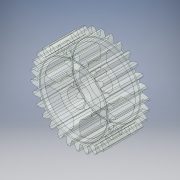
# Autodesk Inventor part: Peça1
Saved by Autodesk Inventor 2019.4 (Build 234330000, 330)
## iProperties
Created: 2020-04-11
Part Number: Peça1
Material: Vidro, fundido, transparente
Document SubType Name: Modeling
Designer: lucas
Density: 2.18 g/cm^3
Appearance: Transparente
Author: lucas
Autodesk Inventor part; units mm, degrees
ref_plane "YZ Plane" through (0, 0, 0) normal (1, 0, 0) x (0, 1, 0)
ref_plane "XZ Plane" through (0, 0, 0) normal (0, 1, 0) x (-1, 0, 0)
ref_plane "XY Plane" through (0, 0, 0) normal (0, 0, 1) x (1, 0, 0)
sketch "Esboço1" plane through (0, 0, 0) normal (0, 0, 1) x (1, 0, 0)
  circle A0 centre (0, 0) radius 35 construction
  arc A1 (-1.094, 31.8562) -> (-3.3459, 37.3504) centre (-14.2896, 29.6565) ccw
  arc A2 (3.3459, 37.3504) -> (1.094, 31.8562) centre (14.2896, 29.6565) ccw
  arc A3 (1.094, 31.8562) -> (-1.094, 31.8562) centre (0, 0) ccw
  arc A4 (6.0221, 31.301) -> (5.0493, 37.1585) centre (-7.3322, 32.0927) ccw
  arc A5 (8.1553, 30.8141) -> (6.0221, 31.301) centre (0, 0) ccw
  arc A6 (11.5732, 35.6695) -> (8.1553, 30.8141) centre (20.5306, 25.7332) ccw
  arc A7 (12.8362, 29.1762) -> (13.1912, 35.1033) centre (-0.007, 32.9196) ccw
  arc A8 (14.8076, 28.2268) -> (12.8362, 29.1762) centre (0, 0) ccw
  arc A9 (19.2203, 32.1999) -> (14.8076, 28.2268) centre (25.742, 20.5196) ccw
  arc A10 (19.0067, 25.5883) -> (20.6717, 31.2879) centre (7.3185, 32.0958) ccw
  arc A11 (20.7174, 24.2241) -> (19.0067, 25.5883) centre (0, 0) ccw
  arc A12 (25.9035, 27.1156) -> (20.7174, 24.2241) centre (29.6626, 14.277) ccw
  arc A13 (24.2241, 20.7174) -> (27.1156, 25.9035) centre (14.277, 29.6626) ccw
  arc A14 (25.5883, 19.0067) -> (24.2241, 20.7174) centre (0, 0) ccw
  arc A15 (31.2879, 20.6717) -> (25.5883, 19.0067) centre (32.0958, 7.3185) ccw
  arc A16 (28.2268, 14.8076) -> (32.1999, 19.2203) centre (20.5196, 25.742) ccw
  arc A17 (29.1762, 12.8362) -> (28.2268, 14.8076) centre (0, 0) ccw
  arc A18 (35.1033, 13.1912) -> (29.1762, 12.8362) centre (32.9196, -0.007) ccw
  arc A19 (30.8141, 8.1553) -> (35.6695, 11.5732) centre (25.7332, 20.5306) ccw
  arc A20 (31.301, 6.0221) -> (30.8141, 8.1553) centre (0, 0) ccw
  arc A21 (37.1585, 5.0493) -> (31.301, 6.0221) centre (32.0927, -7.3322) ccw
  arc A22 (31.8562, 1.094) -> (37.3504, 3.3459) centre (29.6565, 14.2896) ccw
  arc A23 (31.8562, -1.094) -> (31.8562, 1.094) centre (0, 0) ccw
  arc A24 (37.3504, -3.3459) -> (31.8562, -1.094) centre (29.6565, -14.2896) ccw
  arc A25 (31.301, -6.0221) -> (37.1585, -5.0493) centre (32.0927, 7.3322) ccw
  arc A26 (30.8141, -8.1553) -> (31.301, -6.0221) centre (0, 0) ccw
  arc A27 (35.6695, -11.5732) -> (30.8141, -8.1553) centre (25.7332, -20.5306) ccw
  arc A28 (29.1762, -12.8362) -> (35.1033, -13.1912) centre (32.9196, 0.007) ccw
  arc A29 (28.2268, -14.8076) -> (29.1762, -12.8362) centre (0, 0) ccw
  arc A30 (32.1999, -19.2203) -> (28.2268, -14.8076) centre (20.5196, -25.742) ccw
  arc A31 (25.5883, -19.0067) -> (31.2879, -20.6717) centre (32.0958, -7.3185) ccw
  arc A32 (24.2241, -20.7174) -> (25.5883, -19.0067) centre (0, 0) ccw
  arc A33 (27.1156, -25.9035) -> (24.2241, -20.7174) centre (14.277, -29.6626) ccw
  arc A34 (20.7174, -24.2241) -> (25.9035, -27.1156) centre (29.6626, -14.277) ccw
  arc A35 (19.0067, -25.5883) -> (20.7174, -24.2241) centre (0, 0) ccw
  arc A36 (20.6717, -31.2879) -> (19.0067, -25.5883) centre (7.3185, -32.0958) ccw
  arc A37 (14.8076, -28.2268) -> (19.2203, -32.1999) centre (25.742, -20.5196) ccw
  arc A38 (12.8362, -29.1762) -> (14.8076, -28.2268) centre (0, 0) ccw
  arc A39 (13.1912, -35.1033) -> (12.8362, -29.1762) centre (-0.007, -32.9196) ccw
  arc A40 (8.1553, -30.8141) -> (11.5732, -35.6695) centre (20.5306, -25.7332) ccw
  arc A41 (6.0221, -31.301) -> (8.1553, -30.8141) centre (0, 0) ccw
  arc A42 (5.0493, -37.1585) -> (6.0221, -31.301) centre (-7.3322, -32.0927) ccw
  arc A43 (1.094, -31.8562) -> (3.3459, -37.3504) centre (14.2896, -29.6565) ccw
  arc A44 (-1.094, -31.8562) -> (1.094, -31.8562) centre (0, 0) ccw
  arc A45 (-3.3459, -37.3504) -> (-1.094, -31.8562) centre (-14.2896, -29.6565) ccw
  arc A46 (-6.0221, -31.301) -> (-5.0493, -37.1585) centre (7.3322, -32.0927) ccw
  arc A47 (-8.1553, -30.8141) -> (-6.0221, -31.301) centre (0, 0) ccw
  arc A48 (-11.5732, -35.6695) -> (-8.1553, -30.8141) centre (-20.5306, -25.7332) ccw
  arc A49 (-12.8362, -29.1762) -> (-13.1912, -35.1033) centre (0.007, -32.9196) ccw
  arc A50 (-14.8076, -28.2268) -> (-12.8362, -29.1762) centre (0, 0) ccw
  arc A51 (-19.2203, -32.1999) -> (-14.8076, -28.2268) centre (-25.742, -20.5196) ccw
  arc A52 (-19.0067, -25.5883) -> (-20.6717, -31.2879) centre (-7.3185, -32.0958) ccw
  arc A53 (-20.7174, -24.2241) -> (-19.0067, -25.5883) centre (0, 0) ccw
  arc A54 (-25.9035, -27.1156) -> (-20.7174, -24.2241) centre (-29.6626, -14.277) ccw
  arc A55 (-24.2241, -20.7174) -> (-27.1156, -25.9035) centre (-14.277, -29.6626) ccw
  arc A56 (-25.5883, -19.0067) -> (-24.2241, -20.7174) centre (0, 0) ccw
  arc A57 (-31.2879, -20.6717) -> (-25.5883, -19.0067) centre (-32.0958, -7.3185) ccw
  arc A58 (-28.2268, -14.8076) -> (-32.1999, -19.2203) centre (-20.5196, -25.742) ccw
  arc A59 (-29.1762, -12.8362) -> (-28.2268, -14.8076) centre (0, 0) ccw
  arc A60 (-35.1033, -13.1912) -> (-29.1762, -12.8362) centre (-32.9196, 0.007) ccw
  arc A61 (-30.8141, -8.1553) -> (-35.6695, -11.5732) centre (-25.7332, -20.5306) ccw
  arc A62 (-31.301, -6.0221) -> (-30.8141, -8.1553) centre (0, 0) ccw
  arc A63 (-37.1585, -5.0493) -> (-31.301, -6.0221) centre (-32.0927, 7.3322) ccw
  arc A64 (-31.8562, -1.094) -> (-37.3504, -3.3459) centre (-29.6565, -14.2896) ccw
  arc A65 (-31.8562, 1.094) -> (-31.8562, -1.094) centre (0, 0) ccw
  arc A66 (-37.3504, 3.3459) -> (-31.8562, 1.094) centre (-29.6565, 14.2896) ccw
  arc A67 (-31.301, 6.0221) -> (-37.1585, 5.0493) centre (-32.0927, -7.3322) ccw
  arc A68 (-30.8141, 8.1553) -> (-31.301, 6.0221) centre (0, 0) ccw
  arc A69 (-35.6695, 11.5732) -> (-30.8141, 8.1553) centre (-25.7332, 20.5306) ccw
  arc A70 (-29.1762, 12.8362) -> (-35.1033, 13.1912) centre (-32.9196, -0.007) ccw
  arc A71 (-28.2268, 14.8076) -> (-29.1762, 12.8362) centre (0, 0) ccw
  arc A72 (-32.1999, 19.2203) -> (-28.2268, 14.8076) centre (-20.5196, 25.742) ccw
  arc A73 (-25.5883, 19.0067) -> (-31.2879, 20.6717) centre (-32.0958, 7.3185) ccw
  arc A74 (-24.2241, 20.7174) -> (-25.5883, 19.0067) centre (0, 0) ccw
  arc A75 (-27.1156, 25.9035) -> (-24.2241, 20.7174) centre (-14.277, 29.6626) ccw
  arc A76 (-20.7174, 24.2241) -> (-25.9035, 27.1156) centre (-29.6626, 14.277) ccw
  arc A77 (-19.0067, 25.5883) -> (-20.7174, 24.2241) centre (0, 0) ccw
  arc A78 (-20.6717, 31.2879) -> (-19.0067, 25.5883) centre (-7.3185, 32.0958) ccw
  arc A79 (-14.8076, 28.2268) -> (-19.2203, 32.1999) centre (-25.742, 20.5196) ccw
  arc A80 (-12.8362, 29.1762) -> (-14.8076, 28.2268) centre (0, 0) ccw
  arc A81 (-13.1912, 35.1033) -> (-12.8362, 29.1762) centre (0.007, 32.9196) ccw
  arc A82 (-8.1553, 30.8141) -> (-11.5732, 35.6695) centre (-20.5306, 25.7332) ccw
  arc A83 (-6.0221, 31.301) -> (-8.1553, 30.8141) centre (0, 0) ccw
  arc A84 (-5.0493, 37.1585) -> (-6.0221, 31.301) centre (7.3322, 32.0927) ccw
  arc A85 (-3.3459, 37.3504) -> (-5.0493, 37.1585) centre (0, 0) ccw
  arc A86 (-11.5732, 35.6695) -> (-13.1912, 35.1033) centre (0, 0) ccw
  arc A87 (-19.2203, 32.1999) -> (-20.6717, 31.2879) centre (0, 0) ccw
  arc A88 (5.0493, 37.1585) -> (3.3459, 37.3504) centre (0, 0) ccw
  arc A89 (13.1912, 35.1033) -> (11.5732, 35.6695) centre (0, 0) ccw
  arc A90 (20.6717, 31.2879) -> (19.2203, 32.1999) centre (0, 0) ccw
  arc A91 (-25.9035, 27.1156) -> (-27.1156, 25.9035) centre (0, 0) ccw
  arc A92 (-31.2879, 20.6717) -> (-32.1999, 19.2203) centre (0, 0) ccw
  arc A93 (-35.1033, 13.1912) -> (-35.6695, 11.5732) centre (0, 0) ccw
  arc A94 (-37.1585, 5.0493) -> (-37.3504, 3.3459) centre (0, 0) ccw
  arc A95 (-37.3504, -3.3459) -> (-37.1585, -5.0493) centre (0, 0) ccw
  arc A96 (-35.6695, -11.5732) -> (-35.1033, -13.1912) centre (0, 0) ccw
  arc A97 (-32.1999, -19.2203) -> (-31.2879, -20.6717) centre (0, 0) ccw
  arc A98 (-27.1156, -25.9035) -> (-25.9035, -27.1156) centre (0, 0) ccw
  arc A99 (-20.6717, -31.2879) -> (-19.2203, -32.1999) centre (0, 0) ccw
  arc A100 (-13.1912, -35.1033) -> (-11.5732, -35.6695) centre (0, 0) ccw
  arc A101 (-5.0493, -37.1585) -> (-3.3459, -37.3504) centre (0, 0) ccw
  arc A102 (3.3459, -37.3504) -> (5.0493, -37.1585) centre (0, 0) ccw
  arc A103 (11.5732, -35.6695) -> (13.1912, -35.1033) centre (0, 0) ccw
  arc A104 (19.2203, -32.1999) -> (20.6717, -31.2879) centre (0, 0) ccw
  arc A105 (25.9035, -27.1156) -> (27.1156, -25.9035) centre (0, 0) ccw
  arc A106 (31.2879, -20.6717) -> (32.1999, -19.2203) centre (0, 0) ccw
  arc A107 (35.1033, -13.1912) -> (35.6695, -11.5732) centre (0, 0) ccw
  arc A108 (37.1585, -5.0493) -> (37.3504, -3.3459) centre (0, 0) ccw
  arc A109 (37.3504, 3.3459) -> (37.1585, 5.0493) centre (0, 0) ccw
  arc A110 (35.6695, 11.5732) -> (35.1033, 13.1912) centre (0, 0) ccw
  arc A111 (32.1999, 19.2203) -> (31.2879, 20.6717) centre (0, 0) ccw
  arc A112 (27.1156, 25.9035) -> (25.9035, 27.1156) centre (0, 0) ccw
  arc A113 (-6.72, 27.1816) -> (-27.1816, 6.72) centre (0, 0) ccw
  line L0 (-3, 16.9706) -> (-3, 24.2693)
  line L1 (3, -24.2693) -> (3, -16.9706)
  line L2 (3, 16.9706) -> (3, 24.2693)
  arc A114 (27.1816, 6.72) -> (6.72, 27.1816) centre (0, 0) ccw
  arc A115 (14.1421, 5) -> (5, 14.1421) centre (0, 0) ccw
  arc A116 (-5, 14.1421) -> (-14.1421, 5) centre (0, 0) ccw
  line L3 (-3, -24.2693) -> (-3, -16.9706)
  arc A117 (-27.1816, -6.72) -> (-6.72, -27.1816) centre (0, 0) ccw
  arc A118 (6.72, -27.1816) -> (27.1816, -6.72) centre (0, 0) ccw
  arc A119 (-14.1421, -5) -> (-5, -14.1421) centre (0, 0) ccw
  arc A120 (5, -14.1421) -> (14.1421, -5) centre (0, 0) ccw
  line L4 (-24.2693, -3) -> (-16.9706, -3)
  line L5 (16.9706, -3) -> (24.2693, -3)
  line L6 (-24.2693, 3) -> (-16.9706, 3)
  line L7 (16.9706, 3) -> (24.2693, 3)
  arc A121 (-16.9706, 3) -> (-14.1421, 5) centre (-16.9706, 6) ccw
  arc A122 (-5, 14.1421) -> (-3, 16.9706) centre (-6, 16.9706) ccw
  arc A123 (3, 16.9706) -> (5, 14.1421) centre (6, 16.9706) ccw
  arc A124 (14.1421, 5) -> (16.9706, 3) centre (16.9706, 6) ccw
  arc A125 (16.9706, -3) -> (14.1421, -5) centre (16.9706, -6) ccw
  arc A126 (5, -14.1421) -> (3, -16.9706) centre (6, -16.9706) ccw
  arc A127 (-3, -16.9706) -> (-5, -14.1421) centre (-6, -16.9706) ccw
  arc A128 (-14.1421, -5) -> (-16.9706, -3) centre (-16.9706, -6) ccw
  arc A129 (-3, 24.2693) -> (-6.72, 27.1816) centre (-6, 24.2693) ccw
  arc A130 (-27.1816, 6.72) -> (-24.2693, 3) centre (-24.2693, 6) ccw
  arc A131 (-24.2693, -3) -> (-27.1816, -6.72) centre (-24.2693, -6) ccw
  arc A132 (-6.72, -27.1816) -> (-3, -24.2693) centre (-6, -24.2693) ccw
  arc A133 (3, -24.2693) -> (6.72, -27.1816) centre (6, -24.2693) ccw
  arc A134 (27.1816, -6.72) -> (24.2693, -3) centre (24.2693, -6) ccw
  arc A135 (24.2693, 3) -> (27.1816, 6.72) centre (24.2693, 6) ccw
  arc A136 (6.72, 27.1816) -> (3, 24.2693) centre (6, 24.2693) ccw
  arc A137 (-3, 7.4162) -> (3, 7.4162) centre (0, 0) ccw
  line L8 (-3, 10) -> (3, 10)
  line L9 (-3, 10) -> (-3, 7.4162)
  line L10 (3, 10) -> (3, 7.4162)
  point P0 (7.0707, 37.338)
  point P1 (0, 37.5)
  point P2 (7.0707, 39.078)
  point P3 (7.0707, 39.8837)
  point P4 (-27.8388, -3)
  point P5 (3, -27.8388)
  point P6 (3, 27.8388)
  point P7 (-3, 27.8388)
  point P8 (-27.8388, 3)
  point P9 (-3, 14.6969)
  point P10 (3, 14.6969)
  point P11 (27.8388, -3)
  point P12 (27.8388, 3)
  point P13 (14.6969, 3)
  point P14 (-14.6969, -3)
  point P15 (-14.6969, 3)
  point P16 (-3, -27.8388)
  point P17 (3, -14.6969)
  point P18 (14.6969, -3)
  point P19 (-3, -14.6969)
  dimension "d1" = 70
  dimension "d11" = 360
  dimension "d19" = 3
  dimension "d20" = 16
  dimension "d21" = 6
  dimension "d22" = 3
  dimension "d23" = 10
  constraints: 290 point on circle, 138 centre point, 32 tangent, 22 end point, 16 point on line, 15 equal radius, 6 coincident, 1 horizontal, 1 parallel, 1 vertical, 309 other
  measures "d1" diameter of A0
  measures "d19" radius of A121
  measures "d20" diameter of A137
  measures "d21" distance of L8.start L8.end
  measures "d22" horizontal distance of A3.centre L8.end
  measures "d23" distance from line of point (0, 0) L8
extrude "Extrusão1" add sketch "Esboço1" along normal mid plane 30
sketch "Esboço3" plane through (0, 0, 15) normal (0, 0, 1) x (1, 0, 0)
  circle A0 centre (0, 0) radius 30
  dimension "d26" = 60
  constraints: 1 centre point, 1 coincident
  measures "d26" diameter of A0
extrude "Extrusão2" cut sketch "Esboço3" against normal blind 3
mirror "Espelhamento1" about plane through (0, 0, 0) normal (0, 0, 1) of "Extrusão2"
chamfer "Chanfro1" distance 2 angle 45 2 edges at (-30, 0, 12) (-30, 0, -12)
